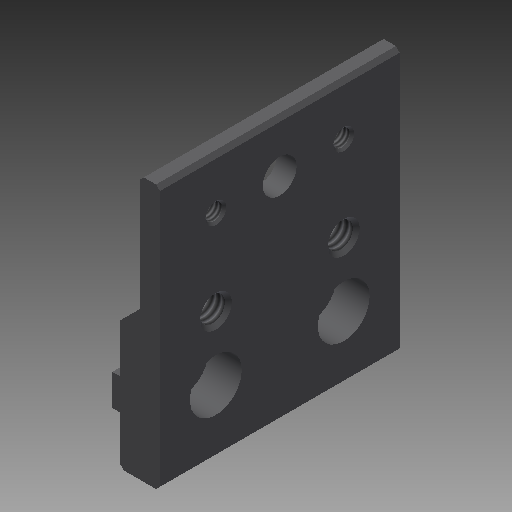
# Autodesk Inventor part: 6760_p
Saved by Autodesk Inventor 2017 (Build 210142000, 142)
## iProperties
Category: PARTsolutions
Company: 8020
Created: 2017-08-19
Part Number: 6760_p
Catalog Web Link: www.cadenas.de
Description: 6760, 6762, 6860, 6862_p-Single UniBearing Bearing
Vendor: 8020
Document SubType Name: Modeling
Designer: psAdmin
Manufacturer: 8020
Mass: 13.6398 g
Surface Area: 68.9754 cm^2
Volume: 13.6398 cm^3
Density: 1 g/cm^3
Material: Generic
Appearance: PSOLRGB-192-192-192
PSOL_IDENT_0: {$CADENAS_DATA\23d-libs\8020\inch\linear_motion\6760.prj},163 {VTYP=3D},{NB=6760_p},{LINA=6760_p},{N
PSOL_IDENT_1: N=6760, 6762, 6860, 6862_p},{DATE=22.08.2012},{GEOMDATE=16.03.2012 00:00:00},{VERSION=},{LINEID=10},
PSOL_IDENT_2: {LINESUBID=-1},{WBVAR=}  {NB=6760_p},{LINA=6760_p},{KT=DUMMY},{PN=6760},{A=0.312},{B=0.156},{C=0.306
PSOL_IDENT_3: },{D=1.165},{E=0.244},{F=1.062},{G=2.062},{H=0.500},{J=1.875},{K=0.437},{K1=0.4375},{L=1.000},{M=0.0
PSOL_IDENT_4: 00},{N=0.000},{R=0.500},{W=.13},{HD=0.257},{CS=0.332},{HD1=0.177},{TH=0.06000},{O=for #8-32},{O1=0.1
PSOL_IDENT_5: 64},{P=1/4-20},{P1=0.2500},{Q=SHCS: 1/4-20x.375\", Double Economy T-Nut: 1/4-20},{Q1=0.40600},{Q2=0.
PSOL_IDENT_6: 257},{Q3=0.260},{S=0.265},{AP=6705},{THRD=1/4-20},{L1=0.375},{TNUT=1/4-20},{NO=1}
NN: 6760, 6762, 6860, 6862_p
NT: Single UniBearing Bearing
NB: 6760_p
NBSYN: $PN._p
LINA: 6760_p
PN: 6760
A: 0.312
B: 0.156
C: 0.306
D: 1.165
E: 0.244
F: 1.062
G: 2.062
H: 0.500
J: 1.875
K: 0.437
K1: 0.4375
L: 1.000
M: 0.000
N: 0.000
R: 0.500
W: .13
HD: 0.257
CS: 0.332
HD1: 0.177
TH: 0.06000
O: for #8-32
O1: 0.164
P: 1/4-20
P1: 0.2500
Q: SHCS: 1/4-20x.375", Double Economy T-Nut: 1/4-20
Q1: 0.40600
Q2: 0.257
Q3: 0.260
S: 0.265
AP: 6705
THRD: 1/4-20
L1: 0.375
TNUT: 1/4-20
NO: 1
SUPPLIER: 8020
ARTICLENO: 6760_p
BOMINFO: 6760_p
CREATOR: CADENAS GmbH
Title: 6760_p
Author: Cadenas PARTsolutions
Comments: Single UniBearing Bearing
Autodesk Inventor part; units mm, degrees
sketch "Sketch_1" plane through (0, 0, 0) normal (0, 0, 1) x (1, 0, 0)
  line L0 (-9.4488, 15.7988) -> (-9.4488, 9.6012)
  line L1 (-9.4488, 9.6012) -> (-7.9248, 9.6012)
  line L2 (-7.9248, 9.6012) -> (-7.9248, 0.762)
  line L3 (-7.9248, 0.762) -> (-7.1628, 0)
  line L4 (-7.1628, 0) -> (-0.762, 0)
  line L5 (-0.762, 0) -> (0, 0.762)
  line L6 (0, 0.762) -> (0, 51.6128)
  line L7 (0, 51.6128) -> (-0.762, 52.3748)
  line L8 (-0.762, 52.3748) -> (-3.2004, 52.3748)
  line L9 (-3.2004, 52.3748) -> (-3.9624, 51.6128)
  line L10 (-3.9624, 51.6128) -> (-3.9624, 29.3624)
  line L11 (-3.9624, 29.3624) -> (-7.9248, 25.4)
  line L12 (-7.9248, 25.4) -> (-7.9248, 15.7988)
  line L13 (-7.9248, 15.7988) -> (-9.4488, 15.7988)
  constraints: 28 end point
extrude "Extrusion1" add sketch "Sketch_1" along normal mid plane 47.625
sketch "Sketch_2" plane through (0, 0, 12.7) normal (0, 0, 1) x (1, 0, 0)
  line L0 (0, 42.291) -> (-3.9624, 42.291)
  line L1 (-3.9624, 42.291) -> (-3.9624, 44.3738)
  line L2 (-3.9624, 44.3738) -> (-3.5331, 43.9445)
  line L3 (-3.5331, 43.9445) -> (-0.4293, 43.9445)
  line L4 (-0.4293, 43.9445) -> (0, 44.3738)
  line L5 (0, 44.3738) -> (0, 42.291)
  line L6 (0, 42.291) -> (-3.9624, 42.291)
  constraints: 14 end point
revolve "Revolution1" cut sketch "Sketch_2" angle 360 about axis through (0, 42.291, 12.7) along (1, 0, 0)
thread "Thread1" size "8-32 UNC" class "2B" standard "ANSI Unified Screw Threads" full length
pattern_linear "Rectangular Pattern1" count 2 spacing 25.4 along (0, 0, -1) of "Revolution1"
sketch "Sketch_4" plane through (0, 0, 12.7) normal (0, 0, 1) x (1, 0, 0)
  line L0 (0, 25.4) -> (-7.9248, 25.4)
  line L1 (-7.9248, 25.4) -> (-7.9248, 28.575)
  line L2 (-7.9248, 28.575) -> (-7.2377, 27.8879)
  line L3 (-7.2377, 27.8879) -> (-0.6871, 27.8879)
  line L4 (-0.6871, 27.8879) -> (0, 28.575)
  line L5 (0, 28.575) -> (0, 25.4)
  line L6 (0, 25.4) -> (-7.9248, 25.4)
  constraints: 14 end point
revolve "Revolution2" cut sketch "Sketch_4" angle 360 about axis through (0, 25.4, 12.7) along (1, 0, 0)
thread "Thread2" size "1/4-20 UNC" class "2B" standard "ANSI Unified Screw Threads" length 6.5507
pattern_linear "Rectangular Pattern2" count 2 spacing 25.4 along (0, 0, -1) of "Revolution2"
sketch "Sketch4" plane through (0, 0.762, 23.8125) normal (1, 0, 0) x (0, 0, -1)
  point P0 (11.1125, 11.938)
hole "Hole1" at (0, 12.7, 12.7) direction (-1, 0, 0) diameter 6.5278 depth 9.4488 counterbore diameter 10.3124 counterbore depth 6.604
pattern_linear "Rectangular Pattern3" count 2 spacing 25.4 along (0, 0, -1) of "Hole1"
sketch "Sketch5" plane through (0, 0.762, 23.8125) normal (1, 0, 0) x (0, 0, -1)
  point P0 (23.8125, 41.529)
hole "Hole2" at (0, 42.291, 0) direction (-1, 0, 0) diameter 6.731 depth 3.9624
ref_plane "to_pad1_XY" through (-3.9624, 42.291, -12.7) normal (1, 0, 0) x (0, 0, -1)
ref_plane "to_pad1_YZ" through (-3.9624, 42.291, -12.7) normal (0, 0, -1) x (0, 1, 0)
ref_plane "to_pad1_ZX" through (-3.9624, 42.291, -12.7) normal (0, 1, 0) x (1, 0, 0)
ref_plane "to_pad2_XY" through (-3.9624, 42.291, -12.7) normal (1, 0, 0) x (0, 0, -1)
ref_plane "to_pad2_YZ" through (-3.9624, 42.291, -12.7) normal (0, 0, -1) x (0, 1, 0)
ref_plane "to_pad2_ZX" through (-3.9624, 42.291, -12.7) normal (0, 1, 0) x (1, 0, 0)
ref_plane "to_profile_XY" through (-7.9248, 12.7, 0) normal (1, 0, 0) x (0, 0, -1)
ref_plane "to_profile_YZ" through (-7.9248, 12.7, 0) normal (0, 0, -1) x (0, 1, 0)
ref_plane "to_profile_ZX" through (-7.9248, 12.7, 0) normal (0, 1, 0) x (1, 0, 0)
ref_plane "to_screw_1_XY" through (-6.604, 12.7, 12.7) normal (1, 0, 0) x (0, 0, -1)
ref_plane "to_screw_1_YZ" through (-6.604, 12.7, 12.7) normal (0, 0, -1) x (0, 1, 0)
ref_plane "to_screw_1_ZX" through (-6.604, 12.7, 12.7) normal (0, 1, 0) x (1, 0, 0)
ref_plane "to_screw_2_XY" through (-6.604, 12.7, -12.7) normal (1, 0, 0) x (0, 0, -1)
ref_plane "to_screw_2_YZ" through (-6.604, 12.7, -12.7) normal (0, 0, -1) x (0, 1, 0)
ref_plane "to_screw_2_ZX" through (-6.604, 12.7, -12.7) normal (0, 1, 0) x (1, 0, 0)
ref_plane "to_screw_3_XY" through (-6.604, 12.7, -12.7) normal (1, 0, 0) x (0, 0, -1)
ref_plane "to_screw_3_YZ" through (-6.604, 12.7, -12.7) normal (0, 0, -1) x (0, 1, 0)
ref_plane "to_screw_3_ZX" through (-6.604, 12.7, -12.7) normal (0, 1, 0) x (1, 0, 0)
ref_plane "to_screw_4_XY" through (-6.604, 12.7, -12.7) normal (1, 0, 0) x (0, 0, -1)
ref_plane "to_screw_4_YZ" through (-6.604, 12.7, -12.7) normal (0, 0, -1) x (0, 1, 0)
ref_plane "to_screw_4_ZX" through (-6.604, 12.7, -12.7) normal (0, 1, 0) x (1, 0, 0)
body "Solid1"
